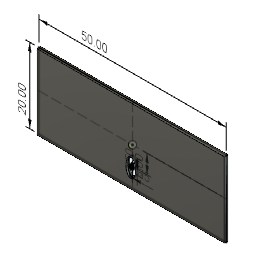
Table_17p1_Problem_11 (Autodesk Fusion 360 design; units mm, degrees)
Autodesk Fusion 360 part; units mm, degrees
sketch "Sketch1" plane through (0, 0, 0) normal (0, 0, 1) x (1, 0, 0)
  line L0 (-250, 100) -> (250, 100)
  line L1 (250, 100) -> (250, -100)
  line L2 (250, -100) -> (-250, -100)
  line L3 (-250, -100) -> (-250, 100)
  line L4 (0, 100) -> (0, -100) construction
  line L5 (-250, 0) -> (250, 0) construction
  ellipse E0 centre (0, -50) end of major axis (0, -25) minor radius 12.5
  line L6 (0, -75) -> (0, -25)
  line L7 (12.5, -50) -> (-12.5, -50)
  dimension "Major_Radius" = 25
  dimension "Minor_Radius" = 12.5
  dimension "Total_Width" = 500
  dimension "Total_Height" = 200
  dimension "Hole_Offset" = 50
  constraint horizontal L0
  constraint vertical L1
  constraint horizontal L2
  constraint vertical L3
  constraint midpoint L0 L4.start
  constraint midpoint L2 L4.end
  constraint midpoint L3 L5.start
  constraint midpoint L1 L5.end
  constraint coincident origin L5
  constraint coincident origin L4
  constraint perpendicular L5 L6
  constraint coincident E0 L6.start
  constraint coincident E0 L6.end
  constraint coincident E0 L7.start
  constraint coincident E0 L7.end
  constraint coincident L4 E0.centre
  measures "Major_Radius" distance of E0
  measures "Total_Width" distance of L0.start L0.end
  measures "Total_Height" distance of L0.start L2.end
  measures "Hole_Offset" distance of L5 L7
extrude "Extrude1" add sketch "Sketch1" along normal mid plane 10
equation "Thickness = 1 cm"
